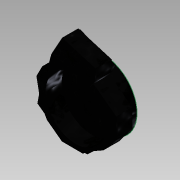
# Autodesk Inventor part: 01_Objektiv
Saved by Autodesk Inventor 2015 (Build 190159000, 159)
## iProperties
Created: 2015-10-11
Part Number: 01_Objektiv
Material: Generisch
Document SubType Name: Modeling
Designer: Bene
Density: 1 g/cm^3
Appearance: Schwarz
Author: Bene
Autodesk Inventor part; units mm, degrees
ref_plane "YZ Plane" through (0, 0, 0) normal (1, 0, 0) x (0, 1, 0)
ref_plane "XZ Plane" through (0, 0, 0) normal (0, 1, 0) x (-1, 0, 0)
ref_plane "XY Plane" through (0, 0, 0) normal (0, 0, 1) x (1, 0, 0)
sketch "Skizze1" plane through (0, 0, 0) normal (0, 1, 0) x (-1, 0, 0)
  line L0 (-198.8627, 53.5938) -> (99.1639, 53.5938) construction
  line L1 (99.1639, 53.5938) -> (99.1639, -114.0462) construction
  line L2 (99.1639, -114.0462) -> (-198.8627, -114.0462) construction
  line L3 (-198.8627, -114.0462) -> (-198.8627, 53.5938) construction
  circle A0 centre (0.0046, 0.0192) radius 18.7265
  line L4 (-9.419, 18.8182) -> (-23.9308, 8.0268)
  line L5 (-23.9308, 8.0268) -> (-23.9308, -2.2349)
  line L6 (-23.9308, -2.2349) -> (-16.3101, -12.64)
  line L7 (-16.3101, -12.64) -> (-10.5238, -15.9026)
  line L8 (-10.5238, -15.9026) -> (-6.65, -19.5009)
  line L9 (-6.65, -19.5009) -> (-5.075, -19.5009)
  line L10 (-5.075, -19.5009) -> (-4.0313, -20.4704)
  line L11 (-4.0313, -20.4704) -> (8.2132, -20.4099)
  line L12 (8.2132, -20.4099) -> (16.9625, -13.9037)
  line L13 (16.9625, -13.9037) -> (18.4985, -11.1795)
  line L14 (18.4985, -11.1795) -> (22.5122, -8.2399)
  line L15 (22.5122, -8.2399) -> (21.5218, -3.0373)
  line L16 (21.5218, -3.0373) -> (23.1766, 5.5058)
  line L17 (23.1766, 5.5058) -> (19.9087, 11.8258)
  line L18 (19.9087, 11.8258) -> (16.0647, 13.9933)
  line L19 (16.0647, 13.9933) -> (14.1168, 21.4913)
  line L20 (14.1168, 21.4913) -> (7.2513, 30.8655)
  line L21 (7.2513, 30.8655) -> (-10.5238, 24.3271)
  line L22 (-10.5238, 24.3271) -> (-10.5238, 20.9548)
  line L23 (-10.5238, 20.9548) -> (-9.419, 18.8182)
  line L24 (-17.1251, -13.5581) -> (-25.1308, -2.6273)
  line L25 (-25.1308, -2.6273) -> (-25.1308, 8.6299)
  line L26 (-25.1308, 8.6299) -> (-10.9532, 19.1727)
  line L27 (-10.9532, 19.1727) -> (-11.7238, 20.6629)
  line L28 (-11.7238, 20.6629) -> (-12.4385, 27.9461)
  line L29 (-12.4385, 27.9461) -> (8.4751, 34.2404)
  line L30 (8.4751, 34.2404) -> (15.2206, 22.0152)
  line L31 (15.2206, 22.0152) -> (17.098, 14.7883)
  line L32 (17.098, 14.7883) -> (20.8101, 12.6952)
  line L33 (20.8101, 12.6952) -> (24.434, 5.6868)
  line L34 (24.434, 5.6868) -> (22.7438, -3.0393)
  line L35 (22.7438, -3.0393) -> (23.8328, -8.7601)
  line L36 (23.8328, -8.7601) -> (19.4166, -11.9945)
  line L37 (19.4166, -11.9945) -> (17.8827, -14.7148)
  line L38 (17.8827, -14.7148) -> (8.6131, -21.608)
  line L39 (8.6131, -21.608) -> (-4.5001, -21.6727)
  line L40 (-4.5001, -21.6727) -> (-5.5463, -20.7009)
  line L41 (-5.5463, -20.7009) -> (-7.1214, -20.7009)
  line L42 (-7.1214, -20.7009) -> (-11.2367, -16.8783)
  line L43 (-11.2367, -16.8783) -> (-17.1251, -13.5581)
  dimension "d4" = 37.453
  dimension "d29" = 42
  dimension "d45" = 1.2
  constraints: 80 end point, 1 centre point, 17 other
  measures "d4" diameter of A0
  measures "d29" distance between parallel lines of L12 L4
  measures "d45" distance between parallel lines of L6 L24
extrude "Extrusion1" add sketch "Skizze1" along normal blind 10 contours L23 L22 L21 L20 L19 L18 L17 L16 L15 L14 L13 L12 L11 L10 L9 L8 L7 L6 L5 L4 | L24 L25 L26 L27 L28 L29 L30 L31 L32 L33 L34 L35 L36 L37 L38 L39 L40 L41 L42 L43
sketch "Skizze2" plane through (0, 10, 0) normal (0, 1, 0) x (1, 0, 0)
  circle A0 centre (-0.0046, -0.0192) radius 18.7265 projected
  line L0 (-9.9482, -31.8575) -> (-12.8321, -24.0172)
  line L1 (-12.8321, -24.0172) -> (9.0572, -15.9655)
  line L2 (9.0572, -15.9655) -> (11.9411, -23.8058)
  line L3 (11.9411, -23.8058) -> (-9.9482, -31.8575)
  line L4 (-7.2513, -30.8655) -> (10.5238, -24.3271) projected
  circle A1 centre (-0.0046, -0.0192) radius 18.7265 projected
  circle A2 centre (-0.0046, -0.0192) radius 21
  point P0 (0, 0)
  point P1 (9.9588, -18.4167)
  point P2 (9.1919, -16.3319)
  point P3 (1.714, -18.6666)
  point P4 (-12.3868, -23.8534)
  dimension "d38" = 42
  constraints: 8 end point, 5 point on line, 2 parallel, 1 centre point, 1 coincident, 1 collinear, 1 perpendicular, 4 other
  measures "d38" diameter of A2
extrude "Extrusion2" add sketch "Skizze2" along normal blind 2.5
sketch "Skizze3" plane through (0, 12.5, 0) normal (0, 1, 0) x (1, 0, 0)
  circle A0 centre (-0.0046, -0.0192) radius 18.7265 projected
  circle A1 centre (-0.0046, -0.0192) radius 21
  point P0 (0, 0)
  dimension "d41" = 42
  constraints: 1 centre point, 1 coincident
  measures "d41" diameter of A1
extrude "Extrusion3" add sketch "Skizze3" along normal blind 4.5 contours A0 | A1
sketch "Skizze4" plane through (-0.0046, 17, 0.0192) normal (0, 1, 0) x (1, 0, 0)
  circle A0 centre (0, 0) radius 21 projected
  point P0 (0.0046, 0.0192)
